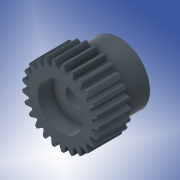
# Autodesk Inventor part: BA011
Saved by Autodesk Inventor 2017 SP1 (Build 210196100, 196)
## iProperties
Created: 2017-06-23
Part Number: BA011
Material: ABS Plastic
Document SubType Name: Modeling
Designer: zallen
Density: 1.06 g/cm^3
Appearance: CR Dark Blue
Author: zallen
Autodesk Inventor part; units mm, degrees
ref_plane "YZ Plane" through (0, 0, 0) normal (1, 0, 0) x (0, 1, 0)
ref_plane "XZ Plane" through (0, 0, 0) normal (0, 1, 0) x (-1, 0, 0)
ref_plane "XY Plane" through (0, 0, 0) normal (0, 0, 1) x (1, 0, 0)
sketch "Sketch1" plane through (0, 0, 0) normal (0, 0, 1) x (1, 0, 0)
  circle A0 centre (0, 0) radius 6
  circle A1 centre (0, 0) radius 18.5
  dimension "d0" = 12
  dimension "d1" = 37
  constraints: 2 centre point, 2 coincident
  measures "d0" diameter of A0
  measures "d1" diameter of A1
extrude "Extrusion1" add sketch "Sketch1" along normal blind 19
sketch "Sketch2" plane through (0, 0, 19) normal (0, 0, 1) x (1, 0, 0)
  line L0 (0, 0) -> (50, 0) construction
  circle A0 centre (0, 0) radius 18.5 projected
  circle A1 centre (0, 0) radius 18.5 projected
  arc A2 (21.9122, 0.65) -> (18.4122, 1.8) centre (15.5154, -12.9176) ccw
  arc A3 (21.9122, -0.65) -> (21.9122, 0.65) centre (1.9228, 0) ccw
  arc A4 (18.4122, -1.8) -> (21.9122, -0.65) centre (15.5154, 12.9176) ccw
  arc A5 (18.4122, -1.8) -> (18.4122, 1.8) centre (0, 0) ccw
  arc A6 (21.0622, 6.0789) -> (17.3861, 6.3224) centre (18.2404, -8.6533) ccw
  arc A7 (21.3855, 4.8198) -> (21.0622, 6.0789) centre (1.8624, 0.4782) ccw
  arc A8 (18.2814, 2.8355) -> (21.3855, 4.8198) centre (11.8154, 16.3703) ccw
  arc A9 (18.2814, 2.8355) -> (17.3861, 6.3224) centre (0, 0) ccw
  arc A10 (18.8887, 11.1259) -> (15.2676, 10.4475) centre (19.8193, -3.8452) ccw
  arc A11 (19.515, 9.9867) -> (18.8887, 11.1259) centre (1.685, 0.9263) ccw
  arc A12 (17.0019, 7.2928) -> (19.515, 9.9867) centre (7.3731, 18.7944) ccw
  arc A13 (17.0019, 7.2928) -> (15.2676, 10.4475) centre (0, 0) ccw
  arc A14 (15.5284, 15.4738) -> (12.1897, 13.9162) centre (20.1529, 1.2045) ccw
  arc A15 (16.4183, 14.5261) -> (15.5284, 15.4738) centre (1.4017, 1.3162) ccw
  arc A16 (14.6541, 11.2919) -> (16.4183, 14.5261) centre (2.4675, 20.0375) ccw
  arc A17 (14.6541, 11.2919) -> (12.1897, 13.9162) centre (0, 0) ccw
  arc A18 (11.1923, 18.8494) -> (8.346, 16.5104) centre (19.2203, 6.1785) ccw
  arc A19 (12.29, 18.1528) -> (11.1923, 18.8494) centre (1.0303, 1.6235) ccw
  arc A20 (11.3856, 14.5815) -> (12.29, 18.1528) centre (-2.5932, 20.0217) ccw
  arc A21 (11.3856, 14.5815) -> (8.346, 16.5104) centre (0, 0) ccw
  arc A22 (6.1531, 21.0406) -> (3.9778, 18.0673) centre (17.0799, 10.7642) ccw
  arc A23 (7.3894, 20.6389) -> (6.1531, 21.0406) centre (0.5942, 1.8287) ccw
  arc A24 (7.4016, 16.9548) -> (7.3894, 20.6389) centre (-7.4909, 18.7478) ccw
  arc A25 (7.4016, 16.9548) -> (3.9778, 18.0673) centre (0, 0) ccw
  arc A26 (0.7272, 21.9098) -> (-0.6403, 18.4889) centre (13.8663, 14.6736) ccw
  arc A27 (2.0246, 21.8282) -> (0.7272, 21.9098) centre (0.1207, 1.919) ccw
  arc A28 (2.9526, 18.2629) -> (2.0246, 21.8282) centre (-11.9179, 16.2959) ccw
  arc A29 (2.9526, 18.2629) -> (-0.6403, 18.4889) centre (0, 0) ccw
  arc A30 (-4.7444, 21.4023) -> (-5.2182, 17.7488) centre (9.7815, 17.6611) ccw
  arc A31 (-3.4675, 21.6459) -> (-4.7444, 21.4023) centre (-0.3603, 1.8887) ccw
  arc A32 (-1.682, 18.4234) -> (-3.4675, 21.6459) centre (-15.5961, 12.82) ccw
  arc A33 (-1.682, 18.4234) -> (-5.2182, 17.7488) centre (0, 0) ccw
  arc A34 (-9.9179, 19.55) -> (-9.4682, 15.8935) centre (5.0821, 19.5388) ccw
  arc A35 (-8.7416, 20.1035) -> (-9.9179, 19.55) centre (-0.8187, 1.7398) ccw
  arc A36 (-6.2109, 17.4263) -> (-8.7416, 20.1035) centre (-18.2943, 8.5387) ccw
  arc A37 (-6.2109, 17.4263) -> (-9.4682, 15.8935) centre (0, 0) ccw
  arc A38 (-14.4682, 16.4693) -> (-13.1233, 13.0395) centre (0.0633, 20.1888) ccw
  arc A39 (-13.4665, 17.298) -> (-14.4682, 16.4693) centre (-1.2256, 1.4815) ccw
  arc A40 (-10.3495, 15.3342) -> (-13.4665, 17.298) centre (-19.8431, 3.7208) ccw
  arc A41 (-10.3495, 15.3342) -> (-13.1233, 13.0395) centre (0, 0) ccw
  arc A42 (-18.1094, 12.3538) -> (-15.9538, 9.3662) centre (-4.9594, 19.5703) ccw
  arc A43 (-17.3453, 13.4055) -> (-18.1094, 12.3538) centre (-1.5556, 1.1302) ccw
  arc A44 (-13.8378, 12.2787) -> (-17.3453, 13.4055) centre (-20.145, -1.3309) ccw
  arc A45 (-13.8378, 12.2787) -> (-15.9538, 9.3662) centre (0, 0) ccw
  arc A46 (-20.6128, 7.4621) -> (-17.7819, 5.1044) centre (-9.6705, 17.7221) ccw
  arc A47 (-20.1342, 8.6708) -> (-20.6128, 7.4621) centre (-1.7878, 0.7078) ccw
  arc A48 (-16.4566, 8.4516) -> (-20.1342, 8.6708) centre (-19.1811, -6.2989) ccw
  arc A49 (-16.4566, 8.4516) -> (-17.7819, 5.1044) centre (0, 0) ccw
  arc A50 (-21.8209, 2.1015) -> (-18.4926, 0.5219) centre (-13.774, 14.7603) ccw
  arc A51 (-21.658, 3.3912) -> (-21.8209, 2.1015) centre (-1.9076, 0.241) ccw
  arc A52 (-18.0414, 4.0935) -> (-21.658, 3.3912) centre (-17.012, -10.8712) ccw
  arc A53 (-18.0414, 4.0935) -> (-18.4926, 0.5219) centre (0, 0) ccw
  arc A54 (-21.658, -3.3912) -> (-18.0414, -4.0935) centre (-17.012, 10.8712) ccw
  arc A55 (-21.8209, -2.1015) -> (-21.658, -3.3912) centre (-1.9076, -0.241) ccw
  arc A56 (-18.4926, -0.5219) -> (-21.8209, -2.1015) centre (-13.774, -14.7603) ccw
  arc A57 (-18.4926, -0.5219) -> (-18.0414, -4.0935) centre (0, 0) ccw
  arc A58 (-20.1342, -8.6708) -> (-16.4566, -8.4516) centre (-19.1811, 6.2989) ccw
  arc A59 (-20.6128, -7.4621) -> (-20.1342, -8.6708) centre (-1.7878, -0.7078) ccw
  arc A60 (-17.7819, -5.1044) -> (-20.6128, -7.4621) centre (-9.6705, -17.7221) ccw
  arc A61 (-17.7819, -5.1044) -> (-16.4566, -8.4516) centre (0, 0) ccw
  arc A62 (-17.3453, -13.4055) -> (-13.8378, -12.2787) centre (-20.145, 1.3309) ccw
  arc A63 (-18.1094, -12.3538) -> (-17.3453, -13.4055) centre (-1.5556, -1.1302) ccw
  arc A64 (-15.9538, -9.3662) -> (-18.1094, -12.3538) centre (-4.9594, -19.5703) ccw
  arc A65 (-15.9538, -9.3662) -> (-13.8378, -12.2787) centre (0, 0) ccw
  arc A66 (-13.4665, -17.298) -> (-10.3495, -15.3342) centre (-19.8431, -3.7208) ccw
  arc A67 (-14.4682, -16.4693) -> (-13.4665, -17.298) centre (-1.2256, -1.4815) ccw
  arc A68 (-13.1233, -13.0395) -> (-14.4682, -16.4693) centre (0.0633, -20.1888) ccw
  arc A69 (-13.1233, -13.0395) -> (-10.3495, -15.3342) centre (0, 0) ccw
  arc A70 (-8.7416, -20.1035) -> (-6.2109, -17.4263) centre (-18.2943, -8.5387) ccw
  arc A71 (-9.9179, -19.55) -> (-8.7416, -20.1035) centre (-0.8187, -1.7398) ccw
  arc A72 (-9.4682, -15.8935) -> (-9.9179, -19.55) centre (5.0821, -19.5388) ccw
  arc A73 (-9.4682, -15.8935) -> (-6.2109, -17.4263) centre (0, 0) ccw
  arc A74 (-3.4675, -21.6459) -> (-1.682, -18.4234) centre (-15.5961, -12.82) ccw
  arc A75 (-4.7444, -21.4023) -> (-3.4675, -21.6459) centre (-0.3603, -1.8887) ccw
  arc A76 (-5.2182, -17.7488) -> (-4.7444, -21.4023) centre (9.7815, -17.6611) ccw
  arc A77 (-5.2182, -17.7488) -> (-1.682, -18.4234) centre (0, 0) ccw
  arc A78 (2.0246, -21.8282) -> (2.9526, -18.2629) centre (-11.9179, -16.2959) ccw
  arc A79 (0.7272, -21.9098) -> (2.0246, -21.8282) centre (0.1207, -1.919) ccw
  arc A80 (-0.6403, -18.4889) -> (0.7272, -21.9098) centre (13.8663, -14.6736) ccw
  arc A81 (-0.6403, -18.4889) -> (2.9526, -18.2629) centre (0, 0) ccw
  arc A82 (7.3894, -20.6389) -> (7.4016, -16.9548) centre (-7.4909, -18.7478) ccw
  arc A83 (6.1531, -21.0406) -> (7.3894, -20.6389) centre (0.5942, -1.8287) ccw
  arc A84 (3.9778, -18.0673) -> (6.1531, -21.0406) centre (17.0799, -10.7642) ccw
  arc A85 (3.9778, -18.0673) -> (7.4016, -16.9548) centre (0, 0) ccw
  arc A86 (12.29, -18.1528) -> (11.3856, -14.5815) centre (-2.5932, -20.0217) ccw
  arc A87 (11.1923, -18.8494) -> (12.29, -18.1528) centre (1.0303, -1.6235) ccw
  arc A88 (8.346, -16.5104) -> (11.1923, -18.8494) centre (19.2203, -6.1785) ccw
  arc A89 (8.346, -16.5104) -> (11.3856, -14.5815) centre (0, 0) ccw
  arc A90 (16.4183, -14.5261) -> (14.6541, -11.2919) centre (2.4675, -20.0375) ccw
  arc A91 (15.5284, -15.4738) -> (16.4183, -14.5261) centre (1.4017, -1.3162) ccw
  arc A92 (12.1897, -13.9162) -> (15.5284, -15.4738) centre (20.1529, -1.2045) ccw
  arc A93 (12.1897, -13.9162) -> (14.6541, -11.2919) centre (0, 0) ccw
  arc A94 (19.515, -9.9867) -> (17.0019, -7.2928) centre (7.3731, -18.7944) ccw
  arc A95 (18.8887, -11.1259) -> (19.515, -9.9867) centre (1.685, -0.9263) ccw
  arc A96 (15.2676, -10.4475) -> (18.8887, -11.1259) centre (19.8193, 3.8452) ccw
  arc A97 (15.2676, -10.4475) -> (17.0019, -7.2928) centre (0, 0) ccw
  arc A98 (21.3855, -4.8198) -> (18.2814, -2.8355) centre (11.8154, -16.3703) ccw
  arc A99 (21.0622, -6.0789) -> (21.3855, -4.8198) centre (1.8624, -0.4782) ccw
  arc A100 (17.3861, -6.3224) -> (21.0622, -6.0789) centre (18.2404, 8.6533) ccw
  arc A101 (17.3861, -6.3224) -> (18.2814, -2.8355) centre (0, 0) ccw
  point P0 (21.9228, 0)
  point P1 (21.234, 5.452)
  point P2 (19.2111, 10.5614)
  point P3 (15.981, 15.0072)
  point P4 (11.7468, 18.51)
  point P5 (6.7745, 20.8498)
  point P6 (1.3765, 21.8795)
  point P7 (-4.1079, 21.5345)
  point P8 (-9.3343, 19.8363)
  point P9 (-13.9741, 16.8918)
  point P10 (-17.7359, 12.8859)
  point P11 (-20.3833, 8.0703)
  point P12 (-21.7499, 2.7477)
  point P13 (-21.7499, -2.7477)
  point P14 (-20.3833, -8.0703)
  point P15 (-17.7359, -12.8859)
  point P16 (-13.9741, -16.8918)
  point P17 (-9.3343, -19.8363)
  point P18 (-4.1079, -21.5345)
  point P19 (1.3765, -21.8795)
  point P20 (6.7745, -20.8498)
  point P21 (11.7468, -18.51)
  point P22 (15.981, -15.0072)
  point P23 (19.2111, -10.5614)
  point P24 (21.234, -5.452)
  dimension "d4" = 50
  dimension "d5" = 15
  dimension "d6" = 3.5
  dimension "d7" = 1.8
  dimension "d8" = 20
  dimension "d10" = 15
  dimension "d12" = 1.8
  dimension "d15" = 360
  dimension "d34" = 1.3
  constraints: 205 point on circle, 100 centre point, 3 coincident, 2 end point, 1 horizontal, 1 point on line, 1 vertical alignment, 324 other
  measures "d4" distance of L0.start L0.end
  measures "d5" radius of A2
  measures "d6" horizontal distance of A2.start A0.start
  measures "d7" distance from line of L0 A0.start
  measures "d8" radius of A3
  measures "d10" radius of A4
  measures "d12" distance from line of L0 A0.end
  measures "d34" distance of A3.start A2.start
extrude "Extrusion2" add sketch "Sketch2" against normal blind 19 contours A0 A2 A3 A4 | A0 A6 A7 A8 | A98 A99 A100 A0 | A0 A10 A11 A12 | A94 A95 A96 A0 | A0 A14 A15 A16 | A90 A91 A92 A0 | A0 A18 A19 A20 | A86 A87 A88 A0 | A0 A22 A23 A24 | A82 A83 A84 A0 | A0 A26 A27 A28 | A78 A79 A80 A0 | A0 A30 A31 A32 | A74 A75 A76 A0 | A0 A34 A35 A36 | A70 A71 A72 A0 | A0 A38 A39 A40 | A66 A67 A68 A0 | A0 A42 A43 A44 | A62 A63 A64 A0 | A0 A46 A47 A48 | A58 A59 A60 A0 | A0 A50 A51 A52 | A54 A55 A56 A0
sketch "Sketch7" plane through (0, 0, 19) normal (0, 0, 1) x (1, 0, 0)
  circle A0 centre (0, 0) radius 13
  dimension "d35" = 26
  constraints: 1 centre point, 1 coincident
  measures "d35" diameter of A0
extrude "Extrusion6" cut sketch "Sketch7" against normal blind 9
sketch "Sketch9" plane through (0, 0, 0) normal (0, 0, -1) x (-1, 0, 0)
  circle A0 centre (0, 0) radius 17.5
  circle A1 centre (0, 0) radius 6 projected
  dimension "d39" = 35
  constraints: 1 centre point, 1 coincident
  measures "d39" diameter of A0
extrude "Extrusion7" add sketch "Sketch9" along normal blind 15
sketch "Sketch10" plane through (0, 0, -15) normal (0, 0, -1) x (-1, 0, 0)
  circle A0 centre (0, 0) radius 13
  dimension "d42" = 26
  constraints: 1 centre point, 1 coincident
  measures "d42" diameter of A0
extrude "Extrusion8" cut sketch "Sketch10" against normal blind 9
body "Solid1"
